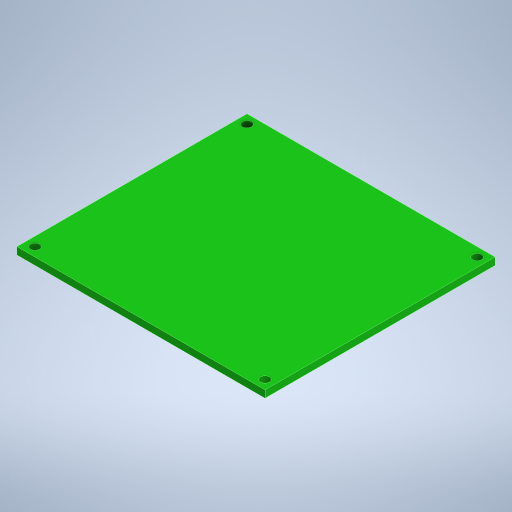
# Autodesk Inventor part: rapoukMotherboardConnectorv0
Saved by Autodesk Inventor 2024 (Build 280153000, 153)
## iProperties
Created: 2024-02-03
Part Number: rapoukMotherboardConnectorv0
Material: Všeobecné
Document SubType Name: Modeling
Designer: Roman Suk
Density: 1 g/cm^3
Appearance: Dark Green
MASSSFP: 400 g
SFP: 4HR
Author: Roman Suk
Autodesk Inventor part; units mm, degrees
ref_plane "YZ Plane" through (0, 0, 0) normal (1, 0, 0) x (0, 1, 0)
ref_plane "XZ Plane" through (0, 0, 0) normal (0, 1, 0) x (-1, 0, 0)
ref_plane "XY Plane" through (0, 0, 0) normal (0, 0, 1) x (1, 0, 0)
sketch "Sketch2" plane through (0, 0, 0) normal (0, 1, 0) x (-1, 0, 0)
  line L0 (-27.5, 25.5) -> (27.5, 25.5)
  line L1 (27.5, 25.5) -> (27.5, -25.5)
  line L2 (27.5, -25.5) -> (-27.5, -25.5)
  line L3 (-27.5, -25.5) -> (-27.5, 25.5)
  line L4 (-27.5, 25.5) -> (27.5, -25.5) construction
  line L5 (27.5, 25.5) -> (-27.5, -25.5) construction
  circle A0 centre (25.5, 23.5) radius 1
  circle A1 centre (25.5, -23.5) radius 1
  circle A2 centre (-25.5, 23.5) radius 1
  circle A3 centre (-25.5, -23.5) radius 1
  line L6 (10, 6) -> (-10, 6)
  line L7 (-10, -6) -> (10, -6)
  line L8 (10, 6) -> (-10, -6) construction
  line L9 (-10, 6) -> (10, -6) construction
  line L10 (10, 6) -> (10, -6)
  line L11 (-10, 6) -> (-10, -6)
  point P0 (0, 0)
  dimension "d2" = 55
  dimension "d3" = 51
  dimension "d4" = 2
  dimension "d5" = 2
  dimension "d6" = 2
  dimension "d9" = 47
  dimension "d12" = 51
  dimension "d17" = 20
  dimension "d18" = 12
  constraints: 24 end point, 4 centre point, 4 midpoint, 3 horizontal, 3 parallel, 3 vertical, 1 perpendicular, 6 other
  measures "d2" distance of L0.start L0.end
  measures "d3" distance between parallel lines of L2 L0
  measures "d4" diameter of A0
  measures "d5" distance from line of L0 A0.centre
  measures "d6" distance from line of L1 A0.centre
  measures "d9" distance of A0.centre A1.centre
  measures "d12" distance of A0.centre A2.centre
  measures "d17" distance of L7.end L7.start
  measures "d18" distance between parallel lines of L6 L7
extrude "Extrusion2" add sketch "Sketch2" along normal blind 1.6 contours L0 L1 L2 L3 | L10 L7 L11 L6
equation "\"d5\" = d4"
equation "\"d6\" = d4"
body "Solid2"
